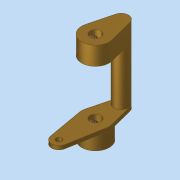
# Autodesk Inventor part: steeringYoke3mmShaft
Saved by Autodesk Inventor 2017 (Build 210142000, 142)
## iProperties
Created: 2016-10-06
Part Number: steeringYoke3mmShaft
Material: Brass, Soft Yellow
Document SubType Name: Modeling
Designer: techn
Density: 8.47 g/cm^3
Appearance: Brass - Satin
Mass: 6.10241 g
Surface Area: 9.16513 cm^2
Volume: 0.720473 cm^3
Author: techn
Autodesk Inventor part; units mm, degrees
ref_plane "XZ Plane" through (0, 0, 0) normal (0, 1, 0) x (-1, 0, 0)
ref_plane "XY Plane" through (0, 0, 0) normal (0, 0, 1) x (1, 0, 0)
sketch "Sketch1" plane through (0, 0, 0) normal (0, 1, 0) x (-1, 0, 0)
  circle A0 centre (0, 0) radius 3.75
  circle A1 centre (0, 0) radius 1.5
  dimension "d0" = 7.5
  dimension "d1" = 3
  constraints: 2 centre point, 2 coincident
  measures "d0" diameter of A0
  measures "d1" diameter of A1
extrude "Extrusion1" add sketch "Sketch1" along normal blind 4
sketch "Sketch2" plane through (0, 4, 0) normal (0, 1, 0) x (1, 0, 0)
  circle A0 centre (0, 0) radius 3.75 projected
  circle A1 centre (0, 0) radius 3.75 projected
  line L0 (0, 0) -> (0, 7)
  circle A2 centre (0, 7) radius 2
  line L1 (-3.6309, 0.9375) -> (-1.9365, 7.5)
  line L2 (1.9365, 7.5) -> (3.6309, 0.9375)
  circle A3 centre (0, 0) radius 1.5 projected
  line L3 (0, 0) -> (0, -10)
  circle A4 centre (0, -10) radius 0.8
  circle A5 centre (0, -10) radius 2
  line L4 (-1.9691, -10.35) -> (-3.6921, -0.6563)
  line L5 (3.6921, -0.6562) -> (1.9691, -10.35)
  dimension "d4" = 7
  dimension "d5" = 4
  dimension "d7" = 10
  dimension "d8" = 1.6
  dimension "d9" = 4
  constraints: 12 end point, 12 point on circle, 8 tangent, 3 centre point, 3 coincident, 2 vertical
  measures "d4" distance of L0.start L0.end
  measures "d5" diameter of A2
  measures "d7" distance of L3.start L3.end
  measures "d8" diameter of A4
  measures "d9" diameter of A5
extrude "Extrusion2" add sketch "Sketch2" along normal blind 1 contours A0 L3 A3 L0 | A0 L0 A2 L2 | L5 A5 L3 A0 | L0 A3 L3 A0 | A0 L1 A2 L0 | A2 | L3 A5 L4 A0 | A5
extrude "Extrusion3" add sketch "Sketch2" along normal blind 16 contours A2
sketch "Sketch3" plane through (0, 20, -7) normal (0, 1, 0) x (1, 0, 0)
  arc A0 (-3.6921, -7.6563) -> (3.6921, -7.6562) centre (0, -7) ccw projected
  arc A1 (3.6309, -6.0625) -> (-3.6309, -6.0625) centre (0, -7) ccw projected
  arc A2 (-3.6309, -6.0625) -> (-3.6921, -7.6563) centre (0, -7) ccw projected
  arc A3 (3.6921, -7.6562) -> (3.6309, -6.0625) centre (0, -7) ccw projected
  circle A4 centre (0, -7) radius 1.5 projected
  line L0 (-1.9365, 0.5) -> (-3.6309, -6.0625) projected
  line L1 (3.6309, -6.0625) -> (1.9365, 0.5) projected
  circle A5 centre (0, 0) radius 2 projected
extrude "Extrusion4" add sketch "Sketch3" along normal blind 1
extrude "Extrusion5" add sketch "Sketch3" along normal blind 5
ref_plane "Work Plane1" through (-3.75, 20, 0) normal (1, 0, 0) x (0, 1, 0)
sketch "Sketch5" plane through (-3.75, 20, 0) normal (1, 0, 0) x (0, 1, 0)
  line L0 (5, 1.5) -> (5, -1.5) projected
  line L1 (0, -1.5) -> (0, 1.5) projected
  line L2 (-15, 1.5) -> (-15, -1.5) projected
  line L3 (-20, -1.5) -> (-20, 1.5) projected
  line L4 (0, 0) -> (5, 0)
  line L5 (-15, 0) -> (-20, 0)
  circle A0 centre (-17.5, 0) radius 1.5
  circle A1 centre (2.5, 0) radius 1.5
  dimension "d19" = 3
  dimension "d20" = 3
  dimension "d27" = 20
  constraints: 5 midpoint, 4 end point, 2 centre point, 1 perpendicular
  measures "d19" diameter of A0
  measures "d20" diameter of A1
  measures "d27" distance of A0.centre A1.centre
extrude "Extrusion6" cut sketch "Sketch5" along normal up to surface
thread "Thread1" size "M3x0.5" class "6H" standard "ANSI Metric M Profile" full length
thread "Thread2" size "M3x0.5" class "6H" standard "ANSI Metric M Profile" full length
body "Solid1"
